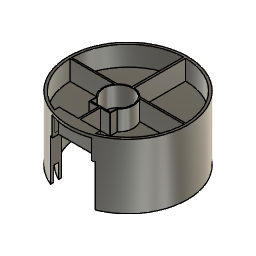
plato final final v2 (Autodesk Fusion 360 design; units mm, degrees)
Autodesk Fusion 360 part; units mm, degrees
sketch "Sketch1" plane through (0, 0, 0) normal (0, 0, 1) x (1, 0, 0)
  circle A0 centre (0, 0) radius 60
  dimension "d1" = 120
  constraint coincident A0.centre origin
  measures "d1" diameter of A0
extrude "Extrude1" add sketch "Sketch1" along normal blind 20
extrude "Extrude2" add 1 faces at (3.7853, -22.4128, 20) along direction (0, 0, 1) blind 5
sketch "Sketch2" plane through (0, 0, 25) normal (0, 0, 1) x (-1, 0, 0)
  circle A0 centre (0, 0) radius 60
  line L0 (0, -60) -> (0, 60)
  line L1 (-60, 0) -> (60, 0)
  line L2 (0, 0) -> (2.5, 0)
  line L3 (2.5, 0) -> (2.5, -70)
  line L4 (2.5, -70) -> (2.5, 65)
  line L5 (2.5, 65) -> (0, 60)
  line L6 (2.5, -70) -> (-2.5, -70)
  line L7 (-2.5, -70) -> (-2.5, 64.2974)
  line L8 (-2.5, 64.2974) -> (2.5, 64.2974)
  line L9 (2.5, 64.2974) -> (2.5, -70)
  line L10 (60, 0) -> (60, -2.5)
  line L11 (60, -2.5) -> (-62.6661, -2.5)
  line L12 (-62.6661, -2.5) -> (-62.6661, 2.5)
  line L13 (-62.6661, 2.5) -> (60, 2.5)
  line L14 (60, 2.5) -> (60, -2.5)
  circle A1 centre (0, 0) radius 55
  dimension "d6" = 2.5
  dimension "d7" = 5
  dimension "d8" = 2.5
  dimension "d9" = 5
  dimension "d10" = 110
  constraint coincident A0 L0.start
  constraint coincident A0 L0.end
  constraint vertical L0
  constraint coincident A0 L1.start
  constraint coincident A0 L1.end
  constraint perpendicular L0 L1
  constraint coincident A0.centre L2.start
  constraint perpendicular L0 L2
  constraint perpendicular L2 L3
  constraint perpendicular L1 L4
  constraint horizontal L6
  constraint vertical L7
  constraint horizontal L8
  constraint vertical L9
  constraint perpendicular L1 L10
  constraint horizontal L11
  constraint vertical L12
  constraint horizontal L13
  constraint vertical L14
  measures "d6" distance of A0.centre L2.end
  measures "d7" distance of L3.end L6.end
  measures "d8" distance of L1.end L10.end
  measures "d9" distance of L10.end L13.end
  measures "d10" diameter of A1
extrude "Extrude3" cut sketch "Sketch2" against normal blind 20 contours L4 L9 L13 A1 | L3 L4 L9 L11 A1 | L7 L13 A1 | L7 L11 A1
sketch "Sketch3" plane through (0, 0, 25) normal (0, 0, 1) x (-1, 0, 0)
  arc A0 (54.9432, 2.5) -> (2.5, 54.9432) centre (0, 0) ccw
  line L0 (54.9432, 2.5) -> (2.5, 2.5)
  line L1 (2.5, 2.5) -> (2.5, 54.9432)
  line L2 (-2.5, 54.9432) -> (-2.5, 2.5)
  line L3 (-2.5, 2.5) -> (-54.9432, 2.5)
  arc A1 (-2.5, 54.9432) -> (-54.9432, 2.5) centre (0, 0) ccw
  line L4 (2.5, -54.9432) -> (2.5, -2.5)
  line L5 (2.5, -2.5) -> (54.9432, -2.5)
  arc A2 (2.5, -54.9432) -> (54.9432, -2.5) centre (0, 0) ccw
  arc A3 (-54.9432, -2.5) -> (-2.5, -54.9432) centre (0, 0) ccw
  line L6 (-54.9432, -2.5) -> (-2.5, -2.5)
  line L7 (-2.5, -2.5) -> (-2.5, -54.9432)
  circle A4 centre (0, 0) radius 60
  circle A5 centre (0, 0) radius 16.5
  circle A6 centre (0, 0) radius 14.5
  dimension "d15" = 33
  dimension "d16" = 29
  constraint coincident A0.centre A1.centre
  constraint concentric A5 A6
  measures "d15" diameter of A5
  measures "d16" diameter of A6
fillet "Fillet1" radius 15 4 edges at (2.5, 2.5, 15) (-2.5, -2.5, 15) (2.5, -2.5, 15) (-2.5, 2.5, 15)
extrude "Extrude4" add sketch "Sketch3" against normal blind 20 contours L0 L5 A5 A6 | L0 L1 A5 A6 | L1 L2 A5 A6 | L2 L3 A5 A6 | L4 L5 A5 A6 | L3 L6 A5 A6 | L4 L7 A5 A6 | L6 L7 A5 A6
sketch "Sketch4" plane through (0, 0, 25) normal (0, 0, 1) x (-1, 0, 0)
  arc A0 (2.5, 17.5) -> (2.5479, 16.3021) centre (17.5, 17.5) ccw
  line L0 (2.5, 17.5) -> (2.5, 54.9432)
  arc A1 (54.9432, 2.5) -> (2.5, 54.9432) centre (0, 0) ccw
  line L1 (54.9432, 2.5) -> (17.5, 2.5)
  arc A2 (16.3021, 2.5479) -> (17.5, 2.5) centre (17.5, 17.5) ccw
  arc A3 (16.3021, 2.5479) -> (2.5479, 16.3021) centre (0, 0) ccw
  arc A4 (-14.2143, 2.8643) -> (-2.8643, 14.2143) centre (-17.5, 17.5) ccw
  arc A5 (-2.8643, 14.2143) -> (-14.2143, 2.8643) centre (0, 0) ccw
  arc A6 (17.5, -2.5) -> (16.3021, -2.5479) centre (17.5, -17.5) ccw
  line L2 (17.5, -2.5) -> (54.9432, -2.5)
  arc A7 (2.5, -54.9432) -> (54.9432, -2.5) centre (0, 0) ccw
  line L3 (2.5, -54.9432) -> (2.5, -17.5)
  arc A8 (2.5479, -16.3021) -> (2.5, -17.5) centre (17.5, -17.5) ccw
  arc A9 (2.5479, -16.3021) -> (16.3021, -2.5479) centre (0, 0) ccw
  arc A10 (-2.8643, -14.2143) -> (-14.2143, -2.8643) centre (-17.5, -17.5) ccw
  arc A11 (-14.2143, -2.8643) -> (-2.8643, -14.2143) centre (0, 0) ccw
  arc A12 (-2.5479, 16.3021) -> (-16.3021, 2.5479) centre (0, 0) ccw
  arc A13 (-17.5, 2.5) -> (-16.3021, 2.5479) centre (-17.5, 17.5) ccw
  line L4 (-17.5, 2.5) -> (-54.9432, 2.5)
  arc A14 (-2.5, 54.9432) -> (-54.9432, 2.5) centre (0, 0) ccw
  line L5 (-2.5, 54.9432) -> (-2.5, 17.5)
  arc A15 (-2.5479, 16.3021) -> (-2.5, 17.5) centre (-17.5, 17.5) ccw
  arc A16 (14.2143, 2.8643) -> (2.8643, 14.2143) centre (0, 0) ccw
  arc A17 (2.8643, 14.2143) -> (14.2143, 2.8643) centre (17.5, 17.5) ccw
  arc A18 (-16.3021, -2.5479) -> (-2.5479, -16.3021) centre (0, 0) ccw
  arc A19 (-2.5, -17.5) -> (-2.5479, -16.3021) centre (-17.5, -17.5) ccw
  line L6 (-2.5, -17.5) -> (-2.5, -54.9432)
  arc A20 (-54.9432, -2.5) -> (-2.5, -54.9432) centre (0, 0) ccw
  line L7 (-54.9432, -2.5) -> (-17.5, -2.5)
  arc A21 (-16.3021, -2.5479) -> (-17.5, -2.5) centre (-17.5, -17.5) ccw
  circle A22 centre (0, 0) radius 60
  arc A23 (2.8643, -14.2143) -> (14.2143, -2.8643) centre (0, 0) ccw
  arc A24 (14.2143, -2.8643) -> (2.8643, -14.2143) centre (17.5, -17.5) ccw
  circle A25 centre (0, 0) radius 14.5
  constraint concentric A1 A25
extrude "Extrude5" cut sketch "Sketch4" against normal blind 20 contours A4 A10 A17 A24 A25
sketch "Sketch5" plane through (0, 0, 25) normal (0, 0, 1) x (-1, 0, 0)
  circle A0 centre (0, 0) radius 14.5
  arc A1 (2.5, 17.5) -> (2.5479, 16.3021) centre (17.5, 17.5) ccw
  line L0 (2.5, 17.5) -> (2.5, 54.9432)
  arc A2 (54.9432, 2.5) -> (2.5, 54.9432) centre (0, 0) ccw
  line L1 (54.9432, 2.5) -> (17.5, 2.5)
  arc A3 (16.3021, 2.5479) -> (17.5, 2.5) centre (17.5, 17.5) ccw
  arc A4 (16.3021, 2.5479) -> (2.5479, 16.3021) centre (0, 0) ccw
  arc A5 (17.5, -2.5) -> (16.3021, -2.5479) centre (17.5, -17.5) ccw
  line L2 (17.5, -2.5) -> (54.9432, -2.5)
  arc A6 (2.5, -54.9432) -> (54.9432, -2.5) centre (0, 0) ccw
  line L3 (2.5, -54.9432) -> (2.5, -17.5)
  arc A7 (2.5479, -16.3021) -> (2.5, -17.5) centre (17.5, -17.5) ccw
  arc A8 (2.5479, -16.3021) -> (16.3021, -2.5479) centre (0, 0) ccw
  arc A9 (-2.5479, 16.3021) -> (-16.3021, 2.5479) centre (0, 0) ccw
  arc A10 (-17.5, 2.5) -> (-16.3021, 2.5479) centre (-17.5, 17.5) ccw
  line L4 (-17.5, 2.5) -> (-54.9432, 2.5)
  arc A11 (-2.5, 54.9432) -> (-54.9432, 2.5) centre (0, 0) ccw
  line L5 (-2.5, 54.9432) -> (-2.5, 17.5)
  arc A12 (-2.5479, 16.3021) -> (-2.5, 17.5) centre (-17.5, 17.5) ccw
  arc A13 (-16.3021, -2.5479) -> (-2.5479, -16.3021) centre (0, 0) ccw
  arc A14 (-2.5, -17.5) -> (-2.5479, -16.3021) centre (-17.5, -17.5) ccw
  line L6 (-2.5, -17.5) -> (-2.5, -54.9432)
  arc A15 (-54.9432, -2.5) -> (-2.5, -54.9432) centre (0, 0) ccw
  line L7 (-54.9432, -2.5) -> (-17.5, -2.5)
  arc A16 (-16.3021, -2.5479) -> (-17.5, -2.5) centre (-17.5, -17.5) ccw
  circle A17 centre (0, 0) radius 60
  line L8 (0, 0) -> (0, 17.5)
  line L9 (0, 0) -> (-17.5, 0)
  line L10 (-17.5, 0) -> (17.5, 0)
  line L11 (0, 17.5) -> (-10, 17.5)
  line L12 (-10, 17.5) -> (10, 17.5)
  line L13 (10, 17.5) -> (10, 13.1244)
  line L14 (-10, 17.5) -> (-10, 13.1244)
  line L15 (10, 13.1244) -> (12, 13.1244)
  line L16 (12, 13.1244) -> (12, 11.3248)
  line L17 (12, 11.3248) -> (12, 19.4998)
  line L18 (12, 19) -> (-12, 19)
  line L19 (-12, 19) -> (-12, 11.3248)
  line L20 (10, 13.1244) -> (10, 10.5)
  line L21 (-10, 13.1244) -> (-10, 13)
  line L22 (-10, 13) -> (-10, 10.5)
  dimension "d21" = 17.5
  dimension "d22" = 35
  dimension "d23" = 8.175
  dimension "d24" = 24
  constraint coincident A0.centre A2.centre
  constraint vertical L8
  constraint perpendicular L8 L9
  constraint parallel L1 L10
  constraint perpendicular L8 L11
  constraint perpendicular L5 L12
  constraint coincident A4 L13.end
  constraint perpendicular L12 L13
  constraint coincident A9 L14.end
  constraint perpendicular L11 L14
  constraint perpendicular L13 L15
  constraint coincident A4 L16.end
  constraint perpendicular L15 L16
  constraint perpendicular L12 L17
  constraint coincident L17 L18.start
  constraint perpendicular L14 L18
  constraint coincident A9 L19.end
  constraint perpendicular L18 L19
  constraint coincident A0 L20.end
  constraint perpendicular L15 L20
  constraint parallel L14 L21
  constraint coincident A0 L22.end
  constraint parallel L14 L22
  measures "d21" distance of A0.centre L9.end
  measures "d22" distance of L9.end L10.end
  measures "d23" distance of L16.end L17.end
  measures "d24" distance of L18.start L18.end
extrude "Extrude6" add sketch "Sketch5" against normal blind 20 contours A4 L15 L16 L17 | L0 L12 L13 L15 L17 L18 | A9 L5 L11 L12 L14 L18 L19
extrude "Extrude7" cut sketch "Sketch5" against normal blind 20 contours A0 A1 A4 L8 L12 L20 | A0 A9 A12 L8 L11 L12 L21 L22
sketch "Sketch6" plane through (0, 0, 0) normal (0, 0, -1) x (1, 0, 0)
  circle A0 centre (0, 0) radius 60
  line L0 (0, 60) -> (0, 50)
  line L1 (0, 50) -> (22.5, 50)
  line L2 (22.5, 50) -> (22.5, 30)
  line L3 (22.5, 50) -> (-22.5, 50)
  line L4 (-22.5, 50) -> (-22.5, 30)
  line L5 (-22.5, 30) -> (22.5, 30)
  line L6 (22.5, 30) -> (22.5, 50)
  dimension "d29" = 22.5
  dimension "d30" = 20
  dimension "d31" = 45
  constraint coincident A0 L0.start
  constraint vertical L0
  constraint perpendicular L0 L1
  constraint perpendicular L1 L2
  constraint horizontal L3
  constraint vertical L4
  constraint horizontal L5
  constraint vertical L6
  measures "d29" distance of L0.end L1.end
  measures "d30" distance of L1.end L2.end
  measures "d31" distance of L1.end L3.end
extrude "Extrude8" add sketch "Sketch6" along normal blind 10
extrude "Extrude9" cut 1 faces at (-7.5, -36.6667, 0) along direction (0, 0, 1) blind 2
sketch "Sketch7" plane through (0, 0, 5) normal (0, 0, 1) x (-1, 0, 0)
  line L0 (10, 10.5) -> (10, 17.5)
  line L1 (10, 17.5) -> (-10, 17.5)
  line L2 (-10, 17.5) -> (-10, 10.5)
  arc A0 (-10, 10.5) -> (10, 10.5) centre (0, 0) ccw
  line L3 (10, 10.5) -> (-10, 10.5)
  line L4 (-10, 10.5) -> (-10, 17.5)
  line L5 (-10, 17.5) -> (10, 17.5)
  line L6 (10, 17.5) -> (10, 10.5)
  constraint horizontal L3
  constraint vertical L4
  constraint horizontal L5
  constraint vertical L6
  constraint coincident L1.end L2.start
  constraint coincident L0.start A0.end
extrude "Extrude10" cut sketch "Sketch7" against normal blind 2100 contours L0 L1 L2 L3 L4 L5 L6
sketch "Sketch8" plane through (0, -30, 0) normal (0, -1, 0) x (1, 0, 0)
  line L0 (-22.5, 2) -> (-22.5, -10)
  line L1 (-22.5, -10) -> (22.5, -10)
  line L2 (22.5, -10) -> (22.5, 2)
  line L3 (22.5, 2) -> (-22.5, 2)
  line L4 (-10, -10) -> (10, -10)
  line L5 (10, -10) -> (10, -5)
  line L6 (10, -5) -> (-10, -5)
  line L7 (-10, -5) -> (-10, -10)
  constraint horizontal L4
  constraint vertical L5
  constraint horizontal L6
  constraint vertical L7
  constraint coincident L1 L4.start
extrude "Extrude11" cut sketch "Sketch8" against normal blind 16 contours L1 L4 L5 L6 L7
extrude "Extrude12" cut 1 faces at (7.5, -50, -2) along direction (0, -1, 0) blind 11
sketch "Sketch9" plane through (0, 0, -10) normal (0, 0, -1) x (1, 0, 0)
  line L0 (22.5, 55.6215) -> (22.5, 30)
  line L1 (22.5, 30) -> (10, 30)
  line L2 (10, 30) -> (10, 10.5)
  line L3 (10, 10.5) -> (-10, 10.5)
  line L4 (-10, 10.5) -> (-10, 30)
  line L5 (-10, 30) -> (-22.5, 30)
  line L6 (-22.5, 30) -> (-22.5, 55.6215)
  arc A0 (-22.5, 55.6215) -> (22.5, 55.6215) centre (0, 0) ccw
  line L7 (-22.5, 30) -> (22.5, 30)
  line L8 (22.5, 30) -> (22.5, 10.5228)
  line L9 (22.5, 10.5228) -> (-22.5, 10.5228)
  line L10 (-22.5, 10.5228) -> (-22.5, 30)
  constraint horizontal L7
  constraint vertical L8
  constraint horizontal L9
  constraint vertical L10
  constraint coincident L5.end L6.start
extrude "Extrude13" cut sketch "Sketch9" against normal blind 12 contours L1 L2 L7 L8 L9 | L2 L4 L7 L9 | L4 L5 L7 L9 L10
sketch "Boceto10" plane through (0, -17.5, 0) normal (0, 1, 0) x (-1, 0, 0)
  line L0 (-10, 2) -> (10, 2)
  line L1 (10, 2) -> (10, 25)
  line L2 (10, 25) -> (-10, 25)
  line L3 (-10, 25) -> (-10, 2)
extrude "Extruir14" add 1 faces at (-1.4159, 12.9498, -10) along direction (0, 0, -1) blind 30
sketch "Boceto12" plane through (0, 0, 0) normal (0, 1, 0) x (1, 0, 0)
  line L0 (0, 40) -> (-20, 40)
  line L1 (-20, 40) -> (-20, -20)
  line L2 (-20, -20) -> (20, -20)
  line L3 (20, -20) -> (20, 40)
  line L4 (20, 40) -> (0, 40)
  dimension "d51" = 20
  dimension "d52" = 60
  dimension "d53" = 40
  constraint horizontal L0
  constraint perpendicular L0 L1
  constraint perpendicular L1 L2
  constraint perpendicular L2 L3
  constraint perpendicular L3 L4
  measures "d51" distance of L0.start L0.end
  measures "d52" distance of L0.end L1.end
  measures "d53" distance of L1.end L2.end
sketch "Boceto13" plane through (0, 0, 2) normal (0, 0, -1) x (1, 0, 0)
  line L0 (-22.5, 55.6215) -> (-22.5, 10.5228)
  line L1 (-22.5, 10.5228) -> (-10, 10.5228)
  line L2 (-10, 10.5228) -> (-10, 17.5)
  line L3 (-10, 17.5) -> (10, 17.5)
  line L4 (10, 17.5) -> (10, 10.5228)
  line L5 (10, 10.5228) -> (22.5, 10.5228)
  line L6 (22.5, 10.5228) -> (22.5, 55.6215)
  arc A0 (22.5, 55.6215) -> (-22.5, 55.6215) centre (0, 0) ccw
  line L7 (0, 60) -> (-20, 60)
  line L8 (-20, 60) -> (-20, 50)
  line L9 (-20, 50) -> (20, 50)
  line L10 (20, 50) -> (20, 60)
  line L11 (20, 60) -> (0, 60)
  dimension "d54" = 20
  constraint midpoint A0 L7.start
  constraint perpendicular L0 L7
  constraint perpendicular L7 L8
  constraint perpendicular L6 L9
  constraint perpendicular L9 L10
  constraint tangent A0 L11
  measures "d54" distance of L7.start L7.end
extrude "Extruir15" cut sketch "Boceto13" against normal blind 20 contours A0 L8 L9 L10
sketch "Boceto15" plane through (0, 0, 5) normal (0, 0, 1) x (-1, 0, 0)
  line L0 (-20, 50) -> (-20, 51.2348)
  arc A0 (-20, 51.2348) -> (-54.9432, 2.5) centre (0, 0) ccw
  line L1 (-54.9432, 2.5) -> (-17.5, 2.5)
  arc A1 (-17.5, 2.5) -> (-16.3021, 2.5479) centre (-17.5, 17.5) ccw
  arc A2 (-12, 11.3248) -> (-16.3021, 2.5479) centre (0, 0) ccw
  line L2 (-12, 11.3248) -> (-12, 19)
  line L3 (-12, 19) -> (-2.5, 19)
  line L4 (-2.5, 19) -> (-2.5, 50)
  line L5 (-2.5, 50) -> (-20, 50)
  line L6 (-20, 50) -> (-20, 49)
  line L7 (-20, 49) -> (-2.5, 49)
  line L8 (-2.5, 50) -> (-20, 50)
  line L9 (20, 50) -> (20, 49)
  line L10 (20, 49) -> (2.3937, 49)
  line L11 (2.3937, 49) -> (2.3937, 50)
  line L12 (2.3937, 50) -> (20, 50)
  constraint coincident L0.start L5.end
  constraint perpendicular L5 L6
  constraint coincident L4 L7.end
  constraint perpendicular L4 L7
  constraint coincident L4.end L5.start
  constraint perpendicular L5 L9
  constraint perpendicular L9 L10
  constraint perpendicular L10 L11
extrude "Extruir16" add sketch "Boceto15" along normal blind 20 contours L4 L5 L6 L7 L8 | L9 L10 L11 L12
sketch "Boceto16" plane through (0, 0, 25) normal (0, 0, 1) x (-1, 0, 0)
  line L0 (2.5, 50) -> (2.5, 54.9432)
  arc A0 (54.9432, 2.5) -> (2.5, 54.9432) centre (0, 0) ccw
  line L1 (54.9432, 2.5) -> (17.5, 2.5)
  arc A1 (16.3021, 2.5479) -> (17.5, 2.5) centre (17.5, 17.5) ccw
  arc A2 (16.3021, 2.5479) -> (12, 11.3248) centre (0, 0) ccw
  line L2 (12, 11.3248) -> (12, 19)
  line L3 (12, 19) -> (2.5, 19)
  line L4 (2.5, 19) -> (2.5, 49)
  line L5 (2.5, 49) -> (20, 49)
  line L6 (20, 49) -> (20, 50)
  line L7 (20, 50) -> (2.5, 50)
  line L8 (10, 17.5) -> (10, 10.5)
  arc A3 (-10, 10.5) -> (10, 10.5) centre (0, 0) ccw
  line L9 (-10, 10.5) -> (-10, 17.5)
  line L10 (-10, 17.5) -> (10, 17.5)
  arc A4 (17.5, -2.5) -> (16.3021, -2.5479) centre (17.5, -17.5) ccw
  line L11 (17.5, -2.5) -> (54.9432, -2.5)
  arc A5 (2.5, -54.9432) -> (54.9432, -2.5) centre (0, 0) ccw
  line L12 (2.5, -54.9432) -> (2.5, -17.5)
  arc A6 (2.5479, -16.3021) -> (2.5, -17.5) centre (17.5, -17.5) ccw
  arc A7 (2.5479, -16.3021) -> (16.3021, -2.5479) centre (0, 0) ccw
  line L13 (-2.5, 19) -> (-12, 19)
  line L14 (-12, 19) -> (-12, 11.3248)
  arc A8 (-12, 11.3248) -> (-16.3021, 2.5479) centre (0, 0) ccw
  arc A9 (-17.5, 2.5) -> (-16.3021, 2.5479) centre (-17.5, 17.5) ccw
  line L15 (-17.5, 2.5) -> (-54.9432, 2.5)
  arc A10 (-2.5, 54.9432) -> (-54.9432, 2.5) centre (0, 0) ccw
  line L16 (-2.5, 54.9432) -> (-2.5, 50)
  line L17 (-2.5, 50) -> (-20, 50)
  line L18 (-20, 50) -> (-20, 49)
  line L19 (-20, 49) -> (-2.5, 49)
  line L20 (-2.5, 49) -> (-2.5, 19)
  arc A11 (-16.3021, -2.5479) -> (-2.5479, -16.3021) centre (0, 0) ccw
  arc A12 (-2.5, -17.5) -> (-2.5479, -16.3021) centre (-17.5, -17.5) ccw
  line L21 (-2.5, -17.5) -> (-2.5, -54.9432)
  arc A13 (-54.9432, -2.5) -> (-2.5, -54.9432) centre (0, 0) ccw
  line L22 (-54.9432, -2.5) -> (-17.5, -2.5)
  arc A14 (-16.3021, -2.5479) -> (-17.5, -2.5) centre (-17.5, -17.5) ccw
  circle A15 centre (0, 0) radius 60
  line L23 (20, 50) -> (20, 51.2348)
  line L24 (2.5, 50) -> (2.5, 54.9432)
  line L25 (-2.5, 50) -> (-20, 50)
  line L26 (-2.5, 50) -> (-2.5, 54.9432)
  line L27 (-20, 50) -> (-2.5, 50)
  line L28 (-20, 50) -> (-20, 51.5)
  constraint coincident L6.end L7.start
  constraint coincident A0 L23.end
  constraint perpendicular L7 L23
  constraint coincident L0.start L7.end
  constraint coincident L0.end A0.end
  constraint coincident L16.end L17.start
  constraint coincident L17.end L18.start
  constraint coincident A10.start L16.start
  constraint perpendicular L17 L28
extrude "Extruir17" add sketch "Boceto16" against normal blind 3 contours L0 A0 L7 L23 L24 | A10 L16 L17 L25 L26 L27 L28
sketch "Boceto17" plane through (0, 0, 5) normal (0, 0, 1) x (-1, 0, 0)
  line L0 (20, 49) -> (2.5, 49)
  line L1 (2.5, 49) -> (2.5, 19)
  line L2 (2.5, 19) -> (12, 19)
  line L3 (12, 19) -> (12, 11.3248)
  arc A0 (16.3021, 2.5479) -> (12, 11.3248) centre (0, 0) ccw
  arc A1 (16.3021, 2.5479) -> (17.5, 2.5) centre (17.5, 17.5) ccw
  line L4 (17.5, 2.5) -> (54.9432, 2.5)
  arc A2 (54.9432, 2.5) -> (20, 51.2348) centre (0, 0) ccw
  line L5 (20, 51.2348) -> (20, 50)
  line L6 (20, 50) -> (20, 49)
  line L7 (20, 49) -> (21, 49)
  line L8 (21, 49) -> (21, 50.8331)
  line L9 (20, 49) -> (20, 51.2348)
  line L10 (-20, 49) -> (-21.5, 49)
  line L11 (-21.5, 49) -> (-21.5, 51.2835)
  line L12 (-21.5, 51.2835) -> (-20, 51.2835)
  line L13 (-20, 51.2835) -> (-20, 49)
  constraint coincident L0.start L6.end
  constraint perpendicular L6 L7
  constraint coincident A2 L8.end
  constraint perpendicular L7 L8
  constraint coincident A2.end L5.start
  constraint horizontal L10
  constraint perpendicular L10 L11
  constraint perpendicular L11 L12
  constraint perpendicular L12 L13
extrude "Extruir18" add sketch "Boceto17" along normal blind 20 contours A2 L5 L6 L7 L8 L9 | L10 L11 L12 L13
sketch "Boceto18" plane through (0, 0, -40) normal (0, 0, -1) x (1, 0, 0)
  line L0 (22.5, 10.5228) -> (10, 10.5228)
  line L1 (10, 10.5228) -> (10, 10.5)
  line L2 (10, 10.5) -> (-10, 10.5)
  line L3 (-10, 10.5) -> (-10, 10.5228)
  line L4 (-10, 10.5228) -> (-22.5, 10.5228)
  line L5 (-22.5, 10.5228) -> (-22.5, 55.6215)
  arc A0 (-22.5, 55.6215) -> (22.5, 55.6215) centre (0, 0) ccw
  line L6 (22.5, 55.6215) -> (22.5, 10.5228)
  circle A1 centre (0, 0) radius 50
  dimension "d63" = 100
  constraint concentric A0 A1
  measures "d63" diameter of A1
extrude "Extruir19" cut sketch "Boceto18" against normal blind 42 contours L0 L1 L2 L3 L4 L5 L6 A1 | L0 L1 L2 L3 L4 L5 L6 A1
sketch "Boceto19" plane through (0, 0, -40) normal (0, 0, -1) x (1, 0, 0)
  arc A0 (-22.5, 44.6514) -> (22.5, 44.6514) centre (0, 0) ccw
  line L0 (-22.5, 44.6514) -> (-22.5, 55.6215)
  arc A1 (-22.5, 55.6215) -> (22.5, 55.6215) centre (0, 0) ccw
  line L1 (22.5, 55.6215) -> (22.5, 44.6514)
  circle A2 centre (0, 0) radius 57.5
  circle A3 centre (0, 0) radius 52.5
  dimension "d66" = 115
  dimension "d67" = 105
  constraint coincident A0.centre A1.centre
  constraint concentric A0 A3
  measures "d66" diameter of A2
  measures "d67" diameter of A3
extrude "Extruir20" cut sketch "Boceto19" against normal blind 15 contours L0 L1 A2 A3 picked at (-25.0293, 49.783)
sketch "Boceto20" plane through (0, 0, -45) normal (0, 0, -1) x (1, 0, 0)
  arc A0 (-22.5, 52.915) -> (22.5, 52.915) centre (0, 0) ccw
  line L0 (22.5, 52.915) -> (22.5, 47.4342)
  arc A1 (-22.5, 47.4342) -> (22.5, 47.4342) centre (0, 0) ccw
  line L1 (-22.5, 47.4342) -> (-22.5, 52.915)
  circle A2 centre (0, 0) radius 60
  dimension "d72" = 120
  constraint concentric A0 A2
  measures "d72" diameter of A2
move_face "MoveFace1" to x (1, 0, 0) y (0, 1, 0) z (0, 0, 1) at (0, 0, -5) 1 faces at (-28.9589, -52.5488, -4.3333)
move_body "Desplazar1" bodies 1 to x (1, 0, 0) y (0, 1, 0) z (0, 0, 1) at (0, 0, 60)
sketch "Boceto21" plane through (0, -50, 0) normal (0, -1, 0) x (1, 0, 0)
  line L0 (20, 82) -> (-2.5, 82)
  line L1 (-2.5, 82) -> (-2.5, 65)
  line L2 (-2.5, 65) -> (-20, 65)
  line L3 (-20, 65) -> (-20, 62)
  line L4 (-20, 62) -> (20, 62)
  line L5 (20, 62) -> (20, 82)
  line L6 (0, 82) -> (20, 82)
  line L7 (20, 82) -> (20, 22)
  line L8 (20, 22) -> (-20, 22)
  line L9 (-20, 22) -> (-20, 82)
  line L10 (-20, 82) -> (0, 82)
  dimension "d79" = 60
  dimension "d80" = 40
  constraint coincident L0 L6.start
  constraint coincident L0.start L5.end
  constraint perpendicular L0 L7
  constraint perpendicular L7 L8
  constraint perpendicular L2 L9
  constraint perpendicular L1 L10
  measures "d79" distance of L0.start L7.end
  measures "d80" distance of L7.end L8.end
extrude "Extruir24" add sketch "Boceto21" along normal blind 1.5
move_body "Desplazar2" bodies 1 to x (1, 0, 0) y (0, 1, 0) z (0, 0, 1) at (0, 0, -53)
sketch "Boceto22" plane through (0, 0, -31) normal (0, 0, -1) x (1, 0, 0)
  line L0 (-20, 50) -> (20, 50)
  line L1 (20, 50) -> (20, 51.5)
  line L2 (20, 51.5) -> (-20, 51.5)
  line L3 (-20, 51.5) -> (-20, 50)
sketch "Boceto23" plane through (0, 0, -45) normal (0, 0, -1) x (1, 0, 0)
sketch "Boceto24" plane through (0, 0, -31) normal (0, 0, -1) x (1, 0, 0)
  line L0 (-20, 50) -> (-11, 50)
  line L1 (20, 50) -> (11, 50)
  line L2 (-11, 50) -> (-11, 51.5)
  line L3 (-20, 50) -> (-20, 51.5)
  line L4 (-20, 51.5) -> (-11, 51.5)
  line L5 (11, 50) -> (11, 51.5)
  line L6 (11, 51.5) -> (20, 51.5)
  line L7 (20, 51.5) -> (20, 50)
  dimension "d85" = 9
  dimension "d86" = 9
  dimension "d87" = 1.5
  dimension "d88" = 1.5
  constraint horizontal L0
  constraint horizontal L1
  constraint perpendicular L0 L2
  constraint perpendicular L0 L3
  constraint perpendicular L1 L5
  constraint perpendicular L2 L6
  constraint perpendicular L1 L7
  measures "d85" distance of L0.start L0.end
  measures "d86" distance of L1.start L1.end
  measures "d87" distance of L0.end L2.end
  measures "d88" distance of L0.start L3.end
sketch "Boceto25" plane through (0, 0, -40) normal (0, 0, 1) x (-1, 0, 0)
  line L0 (20, 51.5) -> (20, 50)
  line L1 (20, 50) -> (-20, 50)
  line L2 (-20, 50) -> (-20, 51.5)
  line L3 (-20, 51.5) -> (20, 51.5)
  circle A0 centre (0, 0) radius 60
  line L4 (20, 50) -> (11, 50)
  line L5 (20, 50) -> (20, 51.5)
  line L6 (20, 51.5) -> (11, 51.5)
  line L7 (11, 50) -> (11, 51.5)
  line L8 (11, 51.5) -> (11, 50)
  line L9 (-20, 50) -> (-11, 50)
  line L10 (-11, 50) -> (-11, 51.5)
  line L11 (-20, 51.5) -> (-20, 50)
  line L12 (22.5, 47.4342) -> (22.5, 52.915)
  arc A1 (-22.5, 52.915) -> (22.5, 52.915) centre (0, 0) ccw
  line L13 (-22.5, 52.915) -> (-22.5, 47.4342)
  arc A2 (-22.5, 47.4342) -> (22.5, 47.4342) centre (0, 0) ccw
  dimension "d89" = 9
  dimension "d90" = 9
  constraint coincident L0.end L1.start
  constraint perpendicular L0 L4
  constraint coincident L0.start L3.end
  constraint coincident L3 L6.end
  constraint perpendicular L0 L6
  constraint coincident L1.end L2.start
  constraint perpendicular L2 L9
  constraint coincident L3 L10.end
  constraint perpendicular L3 L10
  constraint coincident L2.end L3.start
  measures "d89" distance of L0.end L4.end
  measures "d90" distance of L1.end L9.end
move_body "Desplazar3" bodies 1 to x (1, 0, 0) y (0, 1, 0) z (0, 0, 1) at (0, 0, 35)
sketch "Boceto26" plane through (0, 0, -40) normal (0, 0, 1) x (-1, 0, 0)
  line L0 (-11, 50) -> (-11, 45)
  line L1 (-11, 45) -> (11, 45)
  line L2 (11, 45) -> (11, 50)
  line L3 (20, 50) -> (20, 51.5)
  line L4 (20, 51.5) -> (11, 51.5)
  line L5 (11, 51.5) -> (11, 50)
  line L6 (11, 50) -> (20, 50)
  dimension "d95" = 5
  constraint perpendicular L0 L1
  measures "d95" distance of L0.start L0.end
move_body "Desplazar4" bodies 1 to x (1, 0, 0) y (0, 1, 0) z (0, 0, 1) at (0, 0, -45)
move_body "Desplazar5" bodies 1 to x (1, 0, 0) y (0, 1, 0) z (0, 0, 1) at (0, 0, 3)
move_body "Desplazar6" bodies 1 to x (1, 0, 0) y (0, 1, 0) z (0, 0, 1) at (0, 0, 35)
sketch "Boceto27" plane through (0, 0, -45) normal (0, 0, -1) x (1, 0, 0)
  line L0 (-40, 20) -> (-20, 20)
extrude "Extruir29" add 1 faces at (-6.6667, -51.5, 10.3333) along direction (0, -1, 0) blind 1.5
extrude "Extruir30" cut 1 faces at (-6.6667, -53, 10.3333) along direction (0, 1, 0) blind 1.5
extrude "Extruir31" cut 1 faces at (-6.6667, -51.5, 10.3333) along direction (0, 1, 0) blind 1.5
sketch "Boceto28" plane through (0, 0, 60) normal (0, 0, 1) x (-1, 0, 0)
  arc A0 (54.9432, 2.5) -> (21, 50.8331) centre (0, 0) ccw
  line L0 (54.9432, 2.5) -> (17.5, 2.5)
  arc A1 (16.3021, 2.5479) -> (17.5, 2.5) centre (17.5, 17.5) ccw
  arc A2 (16.3021, 2.5479) -> (12, 11.3248) centre (0, 0) ccw
  line L1 (12, 11.3248) -> (12, 19)
  line L2 (12, 19) -> (2.5, 19)
  line L3 (2.5, 19) -> (2.5, 49)
  line L4 (2.5, 49) -> (21, 49)
  line L5 (21, 49) -> (21, 50.8331)
  line L6 (-21.5, 49) -> (-2.5, 49)
  line L7 (-2.5, 49) -> (-2.5, 19)
  line L8 (-2.5, 19) -> (-12, 19)
  line L9 (-12, 19) -> (-12, 11.3248)
  arc A3 (-12, 11.3248) -> (-16.3021, 2.5479) centre (0, 0) ccw
  arc A4 (-17.5, 2.5) -> (-16.3021, 2.5479) centre (-17.5, 17.5) ccw
  line L10 (-17.5, 2.5) -> (-54.9432, 2.5)
  arc A5 (-21.5, 50.6236) -> (-54.9432, 2.5) centre (0, 0) ccw
  line L11 (-21.5, 50.6236) -> (-21.5, 49)
  line L12 (10, 17.5) -> (10, 10.5)
  arc A6 (-10, 10.5) -> (10, 10.5) centre (0, 0) ccw
  line L13 (-10, 10.5) -> (-10, 17.5)
  line L14 (-10, 17.5) -> (10, 17.5)
  arc A7 (17.5, -2.5) -> (16.3021, -2.5479) centre (17.5, -17.5) ccw
  line L15 (17.5, -2.5) -> (54.9432, -2.5)
  arc A8 (2.5, -54.9432) -> (54.9432, -2.5) centre (0, 0) ccw
  line L16 (2.5, -54.9432) -> (2.5, -17.5)
  arc A9 (2.5479, -16.3021) -> (2.5, -17.5) centre (17.5, -17.5) ccw
  arc A10 (2.5479, -16.3021) -> (16.3021, -2.5479) centre (0, 0) ccw
  arc A11 (-16.3021, -2.5479) -> (-2.5479, -16.3021) centre (0, 0) ccw
  arc A12 (-2.5, -17.5) -> (-2.5479, -16.3021) centre (-17.5, -17.5) ccw
  line L17 (-2.5, -17.5) -> (-2.5, -54.9432)
  arc A13 (-54.9432, -2.5) -> (-2.5, -54.9432) centre (0, 0) ccw
  line L18 (-54.9432, -2.5) -> (-17.5, -2.5)
  arc A14 (-16.3021, -2.5479) -> (-17.5, -2.5) centre (-17.5, -17.5) ccw
  circle A15 centre (0, 0) radius 60
  line L19 (0, 0) -> (0, 10)
  circle A16 centre (0, 10) radius 14.5
  line L20 (10, 17.5) -> (10, 27.5)
  line L21 (-10, 17.5) -> (-10, 27.5)
  line L22 (10, 27.5) -> (-10, 27.5)
  line L23 (12, 19) -> (12, 29.5)
  line L24 (12, 29.5) -> (-12, 29.5)
  line L25 (-12, 29.5) -> (-12, 19)
  dimension "d116" = 10
  dimension "d117" = 29
  dimension "d118" = 10
  dimension "d119" = 10
  constraint coincident A0.centre A2.centre
  constraint vertical L19
  constraint coincident L19.end A16.centre
  constraint coincident L12.start L14.end
  constraint perpendicular L2 L20
  constraint coincident L13.end L14.start
  constraint perpendicular L14 L21
  constraint coincident L1.end L2.start
  constraint perpendicular L22 L23
  constraint perpendicular L9 L24
  constraint coincident L8.end L9.start
  constraint perpendicular L8 L25
  measures "d116" distance of A0.centre L19.end
  measures "d117" diameter of A16
  measures "d118" distance of L12.start L20.end
  measures "d119" distance of L13.end L21.end
sketch "Boceto29" plane through (0, 0, 60) normal (0, 0, 1) x (-1, 0, 0)
  circle A0 centre (0, 0) radius 60
  dimension "d120" = 120
  constraint coincident A0.centre origin
  measures "d120" diameter of A0
extrude "Extruir32" add sketch "Boceto28" against normal blind 20 contours A0 L0 A1 A2 L1 L3 L4 L5 A16 L23 L24 | L12 A6 L13 L14 A16 | L3 A16 L20 L22 | L6 L7 L9 A3 A4 L10 A5 L11 A16 L24 L25 | L2 L3 A16 L20 | L7 A16 L21 L22 | L7 L8 A16 L21 | A7 L15 A8 L16 A9 A10 | A11 A12 L17 A13 L18 A14
extrude "Extruir33" add sketch "Boceto28" against normal blind 20 contours A2 L1 A16 | L2 L3 A16 L20 L22 L23 L24 | A6 A16 | L7 L8 A16 L21 L22 L24 L25 | L9 A3 A16
extrude "Extruir34" cut sketch "Boceto28" against normal blind 20 contours A2 L1 L2 L12 A6 A16 L20 | A2 L1 A16 | L12 A6 L13 L14 A16 | L3 A16 L20 L22 | L3 L7 A16 L22 | L8 L9 A3 A6 L13 A16 L21 | L2 L3 A16 L20 | L2 L3 L7 L8 L14 A16 L20 L21 | L7 A16 L21 L22 | L2 A16 L20 | L9 A3 A16 | L7 L8 A16 L21 | L8 A16 L21
sketch "Boceto30" plane through (0, 0, 40) normal (0, 0, 1) x (-1, 0, 0)
  line L0 (10, 17.5) -> (10, 10.5)
  line L1 (10, 10.5) -> (-10, 10.5)
  line L2 (-10, 10.5) -> (-10, 17.5)
  line L3 (-10, 17.5) -> (10, 17.5)
  arc A0 (-10, 20.5) -> (10, 20.5) centre (0, 10) ccw
  line L4 (10, 20.5) -> (10, 27.5)
  line L5 (10, 27.5) -> (-10, 27.5)
  line L6 (-10, 27.5) -> (-10, 20.5)
  line L7 (10, 27.5) -> (-10, 27.5)
  line L8 (-10, 27.5) -> (-10, 35)
  line L9 (-10, 35) -> (10, 35)
  line L10 (10, 35) -> (10, 27.5)
  constraint horizontal L7
  constraint vertical L8
  constraint horizontal L9
  constraint vertical L10
  constraint coincident L4.end L5.start
sketch "Boceto31" plane through (0, 0, 40) normal (0, 0, 1) x (-1, 0, 0)
  line L0 (10, 17.5) -> (10, 10.5)
  line L1 (10, 10.5) -> (-10, 10.5)
  line L2 (-10, 10.5) -> (-10, 17.5)
  line L3 (-10, 17.5) -> (10, 17.5)
  arc A0 (-10, 20.5) -> (10, 20.5) centre (0, 10) ccw
  line L4 (10, 20.5) -> (10, 27.5)
  line L5 (10, 27.5) -> (-10, 27.5)
  line L6 (-10, 27.5) -> (-10, 20.5)
  line L7 (-10, 10.5) -> (10, 10.5)
  line L8 (10, 10.5) -> (10, 17.5)
  line L9 (10, 17.5) -> (-10, 17.5)
  line L10 (-10, 17.5) -> (-10, 10.5)
  constraint horizontal L7
  constraint vertical L8
  constraint horizontal L9
  constraint vertical L10
  constraint coincident L0.start L3.end
  constraint coincident L1.end L2.start
sketch "Boceto32" plane through (0, 0, 40) normal (0, 0, 1) x (-1, 0, 0)
  line L0 (10, 17.5) -> (10, 10.5)
  line L1 (10, 10.5) -> (-10, 10.5)
  line L2 (-10, 10.5) -> (-10, 17.5)
  line L3 (-10, 17.5) -> (10, 17.5)
  arc A0 (-10, 20.5) -> (10, 20.5) centre (0, 10) ccw
  line L4 (10, 20.5) -> (10, 27.5)
  line L5 (10, 27.5) -> (-10, 27.5)
  line L6 (-10, 27.5) -> (-10, 20.5)
  line L7 (10, 17.5) -> (-10, 17.5)
  line L8 (-10, 17.5) -> (-10, 10.5)
  line L9 (-10, 10.5) -> (10, 10.5)
  line L10 (10, 10.5) -> (10, 17.5)
  constraint horizontal L7
  constraint vertical L8
  constraint horizontal L9
  constraint vertical L10
  constraint coincident L1.end L2.start
  constraint coincident L0.start L3.end
sketch "Boceto33" plane through (0, 0, 60) normal (0, 0, 1) x (-1, 0, 0)
  line L0 (10, 27.5) -> (10, 20.5)
  arc A0 (-10, 20.5) -> (10, 20.5) centre (0, 10) ccw
  line L1 (-10, 20.5) -> (-10, 27.5)
  line L2 (-10, 27.5) -> (10, 27.5)
  circle A1 centre (0, 0) radius 60
  line L3 (-10, 20.5) -> (10, 20.5)
  constraint coincident A0.start L1.start
  constraint coincident L0.end A0.end
extrude "Extruir35" cut sketch "Boceto33" against normal blind 50 contours L0 L1 L2 L3
extrude "Extruir36" add sketch "Boceto28" against normal blind 23 contours L12 A6 L13 L14 A16
extrude "Extruir37" cut sketch "Boceto28" against normal blind 20 contours L12 A6 L13 L14 A16
sketch "Boceto34" plane through (0, 0, 60) normal (0, 0, 1) x (-1, 0, 0)
  arc A0 (-10, 20.5) -> (10, 20.5) centre (0, 10) ccw
  line L0 (-10, 20.5) -> (-10, 27.5)
  line L1 (-10, 27.5) -> (10, 27.5)
  line L2 (10, 27.5) -> (10, 20.5)
  circle A1 centre (0, 0) radius 60
sketch "Boceto35" plane through (0, 0, 60) normal (0, 0, 1) x (-1, 0, 0)
  arc A0 (-10, 20.5) -> (10, 20.5) centre (0, 10) ccw
  line L0 (-10, 20.5) -> (-10, 27.5)
  line L1 (-10, 27.5) -> (10, 27.5)
  line L2 (10, 27.5) -> (10, 20.5)
  circle A1 centre (0, 0) radius 60
  circle A2 centre (0, 0) radius 55
  circle A3 centre (0, 0) radius 55
  dimension "d133" = 110
  measures "d133" diameter of A2
sketch "Boceto36" plane through (0, 0, 60) normal (0, 0, 1) x (-1, 0, 0)
  arc A0 (-10, 20.5) -> (10, 20.5) centre (0, 10) ccw
  line L0 (-10, 20.5) -> (-10, 27.5)
  line L1 (-10, 27.5) -> (10, 27.5)
  line L2 (10, 27.5) -> (10, 20.5)
  circle A1 centre (0, 0) radius 60
  circle A2 centre (0, 0) radius 57.5
  line L3 (0, 0) -> (57.5, 0)
  line L4 (0, 0) -> (0, 57.5)
  line L5 (0, 0) -> (-57.5, 0)
  line L6 (0, 0) -> (0, -57.5)
  circle A3 centre (0, 10) radius 15.5242
  line L7 (10.5065, 21.4286) -> (-10.5065, 21.4286)
  line L8 (-10.5065, 28.75) -> (10.5065, 28.75)
  line L9 (10.5065, 28.75) -> (10.5065, 21.4286)
  line L10 (57.5, 0) -> (11.8743, 0)
  line L11 (-10.5065, 28.75) -> (-10.5065, 21.4286)
  line L12 (-57.4952, -0.7415) -> (-11.208, -0.7415)
  line L13 (-0.6576, -5.5102) -> (-0.6576, -57.4962)
  line L14 (12.6459, 0.9955) -> (57.4914, 0.9955)
  line L15 (20.5303, 53.7099) -> (20.5303, 49)
  line L16 (20.5303, 49) -> (-21, 49)
  line L17 (-21, 49) -> (-21, 53.528)
  line L18 (-0.7877, 28.75) -> (-0.7877, 49)
  line L19 (0.9305, 28.75) -> (0.9305, 49)
  line L20 (11.3739, -0.5657) -> (57.4972, -0.5657)
  line L21 (1.4539, -5.4559) -> (1.4539, -57.4816)
  line L22 (-12.8882, 1.3458) -> (-57.4842, 1.3458)
  line L23 (12.6459, 0.9955) -> (-57.4914, 0.9955)
  dimension "d134" = 115
  constraint concentric A1 A2
  constraint coincident A1.centre A2.centre
  constraint coincident A2 L3.end
  constraint horizontal L3
  constraint coincident A2 L4.end
  constraint perpendicular L3 L4
  constraint coincident A2 L5.end
  constraint perpendicular L4 L5
  constraint coincident A2 L6.end
  constraint perpendicular L3 L6
  constraint concentric A0 A3
  constraint coincident A3 L7.start
  constraint coincident A3 L7.end
  constraint perpendicular L0 L7
  constraint perpendicular L4 L8
  constraint perpendicular L7 L9
  constraint coincident L3 L10.end
  constraint coincident A3 L10.end
  constraint perpendicular L7 L11
  constraint coincident A2 L12.start
  constraint coincident A3 L12.end
  constraint parallel L5 L12
  constraint coincident A3 L13.start
  constraint coincident A2 L13.end
  constraint perpendicular L5 L13
  constraint coincident A3 L14.start
  constraint coincident A2 L14.end
  constraint perpendicular L13 L14
  constraint coincident A2 L15.start
  constraint perpendicular L14 L15
  constraint perpendicular L4 L16
  constraint coincident A2 L17.end
  constraint perpendicular L16 L17
  constraint coincident L8 L18.start
  constraint coincident L16 L18.end
  constraint perpendicular L16 L18
  constraint coincident L8 L19.start
  constraint coincident L16 L19.end
  constraint perpendicular L16 L19
  constraint coincident A3 L20.start
  constraint coincident A2 L20.end
  constraint parallel L10 L20
  constraint coincident A3 L21.start
  constraint coincident A2 L21.end
  constraint perpendicular L20 L21
  constraint coincident A3 L22.start
  constraint coincident A2 L22.end
  constraint perpendicular L21 L22
  constraint coincident A2 L23.end
  constraint parallel L22 L23
  measures "d134" diameter of A2
extrude "Extruir38" cut sketch "Boceto36" against normal blind 20 contours A2 A3 L22 L23 | A2 L5 A3 L23 | A2 A3 L8 L11 L16 L17 L18 L22 | A2 L6 A3 L21 | A2 A3 L12 L13 | A2 A3 L8 L9 L14 L15 L16 L19 | A2 L3 A3 L10 L20 | A2 A3 L20 L21 | L4 L8 L16 L19
extrude "Extruir39" add sketch "Boceto36" against normal blind 20 contours A2 A3 L22 L23 | A2 L5 A3 L23 | A2 L6 A3 L21 | A2 L3 A3 L10 L20 | L4 L8 L16 L19
extrude "Extruir40" cut sketch "Boceto36" against normal blind 20 contours A2 A3 L22 L23
equation "d21 = ( 35 / 2 ) * 1 mm"
equation "d23 = 6.175 mm + 2 mm"
equation "d29 = ( 45 / 2 ) * 1 mm"
